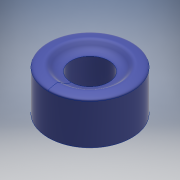
# Autodesk Inventor part: Urethane 97mm
Saved by Autodesk Inventor 2018 (Build 220112000, 112)
## iProperties
Created: 2017-09-13
Part Number: Urethane 97mm
Material: Plastic, Opaque Black
Document SubType Name: Modeling
Designer: Rus
Density: 0.952 g/cm^3
Appearance: Smooth - Black
Author: Rus
Autodesk Inventor part; units mm, degrees
ref_plane "YZ Plane" through (0, 0, 0) normal (1, 0, 0) x (0, 1, 0)
ref_plane "XZ Plane" through (0, 0, 0) normal (0, 1, 0) x (-1, 0, 0)
ref_plane "XY Plane" through (0, 0, 0) normal (0, 0, 1) x (1, 0, 0)
sketch "Sketch1" plane through (0, 0, 0) normal (1, 0, 0) x (0, 1, 0)
  spline S0 degree 3 poles (-21.8, 19) (-21.8911, 18.9704) (-23.5777, 19.1791) (-27.2185, 19.809) (-31.5857, 22.2001) (-34.2433, 25.5665) (-37.0578, 26.9358) (-39.8917, 26.6297) (-42.8949, 26.0623) (-45.8688, 25.4606) (-48.1326, 24.4893) (-48.5091, 23.6382) (-48.5, 23.25) knots 0 0 0 0 0.008681 0.173507 0.363577 0.490264 0.601083 0.655384 0.772555 0.905868 0.967377 1 1 1 1
  line L0 (-48.5, -23.25) -> (-48.5, 23.25)
  arc A0 (-48.5, -23.25) -> (-43.72, -26.1) centre (-43.3877, -20.1092) ccw
  line L1 (-42.92, -26.1) -> (-43.72, -26.1)
  spline S1 degree 3 poles (-36.22, -26.1708) (-32.3391, -21.8472) (-27.5324, -19.457) (-21.8, -19) knots 0 0 0 0 1 1 1 1
  line L2 (-21.8, 19) -> (-21.8, -19)
  line L3 (0, 0) -> (-21.8, 0)
  line L4 (-21.8, 19) -> (-21.8, -19)
  line L5 (-36.22, -26.1708) -> (-37.22, -26.1708)
  line L6 (-37.22, -26.1708) -> (-37.22, -20.4971)
  line L7 (-37.22, -20.4971) -> (-41.92, -20.4971)
  line L8 (-42.92, -26.1) -> (-41.92, -26.1)
  line L9 (-41.92, -26.1) -> (-41.92, -20.4971)
  line L10 (0, 0) -> (0, -18.1714)
  dimension "d0" = 21.8
  dimension "d1" = 38
  dimension "d2" = 1
  dimension "d3" = 1
  dimension "d4" = 4.7
  dimension "d5" = 5.6737
  dimension "d6" = 6
  dimension "d7" = 48.5
  constraints: 22 end point, 3 perpendicular, 2 horizontal, 2 point on circle, 1 centre point, 1 midpoint, 1 vertical, 5 other
  measures "d0" distance of L3.start L3.end
  measures "d1" distance of L4.start L4.end
  measures "d2" distance of L5.start L5.end
  measures "d3" distance of L1.start L8.end
  measures "d4" distance of L6.end L7.end
  measures "d5" distance of L5.end L6.end
  measures "d6" radius of A0
  measures "d7" distance from line of L0 point (0, 0)
revolve "Revolution1" add sketch "Sketch1" angle 360 about axis through (0, 0, 0) along (0, 0, -1)
body "Solid1"
